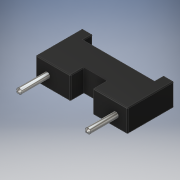
# Autodesk Inventor part: IC_Sockel_2P_2
Saved by Autodesk Inventor 2017 SP1 (Build 210196100, 196)
## iProperties
Part Number: IC_Sockel_2P_2
Material: Generisch
Document SubType Name: Modeling
Designer: Alex
Density: 1 g/cm^3
Appearance: Vorgabe
Author: Alex
Autodesk Inventor part; units mm, degrees
sketch "Skizze1" plane through (0, 0, 0) normal (0, 0, 1) x (1, 0, 0)
  line L0 (0, 0) -> (5.08, 0)
  line L1 (5.08, 0) -> (5.08, 5.16)
  line L2 (5.08, 5.16) -> (0, 5.16)
  line L3 (0, 5.16) -> (0, 0)
  dimension "d0" = 5.08
  dimension "d1" = 5.16
  constraints: 8 end point, 2 parallel, 1 horizontal, 1 perpendicular
  measures "d0" distance of L2.end L1.end
  measures "d1" distance of L1.end L0.end
extrude "Extrusion1" add sketch "Skizze1" against normal blind 2.54
sketch "Skizze2" plane through (0, 0, 0) normal (0, -1, 0) x (1, 0, 0)
  circle A0 centre (3.81, -1.27) radius 0.3
  line L0 (0, 0) -> (0, -2.54) projected
  line L1 (0, -2.54) -> (5.08, -2.54) projected
  dimension "d4" = 0.6
  dimension "d5" = 3.81
  dimension "d7" = 1.27
  constraints: 1 centre point
  measures "d4" diameter of A0
  measures "d5" distance from line of L0 A0.centre
  measures "d7" distance from line of L1 A0.centre
extrude "Extrusion2" add sketch "Skizze2" along normal blind 3.3
sketch "Skizze3" plane through (0, 5.16, 0) normal (0, 1, 0) x (1, 0, 0)
  line L0 (1.935, 2.02) -> (3.935, 2.02)
  line L1 (3.935, 2.02) -> (3.935, 0.52)
  line L2 (3.935, 0.52) -> (1.935, 0.52)
  line L3 (1.935, 0.52) -> (1.935, 2.02)
  line L4 (5.08, 0) -> (5.08, 2.54) projected
  line L5 (5.08, 0) -> (0, 0) projected
  dimension "d10" = 2
  dimension "d11" = 1.5
  dimension "d12" = 1.145
  dimension "d13" = 0.52
  constraints: 8 end point, 2 parallel, 1 horizontal, 1 perpendicular
  measures "d10" distance of L1.end L2.end
  measures "d11" distance of L0.end L1.end
  measures "d12" distance between parallel lines of L4 L1
  measures "d13" distance between parallel lines of L5 L2
extrude "Extrusion3" cut sketch "Skizze3" against normal blind 2
sketch "Skizze4" plane through (0, 3.16, 0) normal (0, 1, 0) x (1, 0, 0)
  line L0 (3.935, 2.02) -> (3.935, 0.52) projected
  line L1 (3.935, 0.52) -> (1.935, 0.52) projected
  line L2 (3.935, 2.02) -> (3.435, 2.02)
  line L3 (3.435, 2.02) -> (3.435, 0.52)
  line L4 (3.435, 0.52) -> (3.935, 0.52)
  line L5 (3.935, 0.52) -> (3.935, 2.02)
  point P0 (0, 0)
  dimension "d16" = 0.5
  constraints: 8 end point, 2 parallel, 1 horizontal, 1 perpendicular, 1 point on line
  measures "d16" distance of L4.end L3.end
extrude "Extrusion4" cut sketch "Skizze4" against normal blind 1
chamfer "Fase1" distance 0.5 angle 45 1 edges at (3.435, 3.16, -1.27)
ref_plane "Arbeitsebene1" through (0, 5.16, -2.54) normal (0, 1, 0) x (1, 0, 0)
ref_plane "Arbeitsebene2" through (0, 0, -2.54) normal (-1, 0, 0) x (0, 0, 1)
fillet "Rundung1" radius 1 1 edges at (2.935, 3.16, -1.27)
fillet "Rundung2" radius 0.5 1 edges at (3.435, 2.66, -1.27)
chamfer "Fase2" distance 0.2 angle 45 1 edges at (3.51, -3.3, -1.27)
mirror "Spiegeln1" about plane through (0, 0, -2.54) normal (-1, 0, 0) of "Extrusion1", "Extrusion2", "Extrusion3", "Extrusion4", "Fase1", "Rundung1", "Rundung2", "Fase2"
pattern_of_one "Rechteckige Anordnung1"
sketch "Skizze5" plane through (0, 5.16, -2.54) normal (0, 1, 0) x (1, 0, 0)
  line L0 (3.935, -2.54) -> (-3.935, -2.54)
  line L1 (-3.935, -2.54) -> (-3.935, 0)
  line L2 (-3.935, 0) -> (3.935, 0)
  line L3 (3.935, 0) -> (3.935, -2.54)
  line L4 (5.08, -2.54) -> (-5.08, -2.54) projected
  line L5 (-3.935, -2.02) -> (-3.935, -0.52) projected
  line L6 (3.935, -0.52) -> (3.935, -2.02) projected
  point P0 (0, -2.54)
  point P1 (0, -2.54)
  dimension "versenkung_Z" = 2.54
  constraints: 8 end point, 2 collinear, 2 midpoint, 2 parallel, 1 perpendicular
  measures "versenkung_Z" distance of L0.end L1.end
extrude "Extrusion5" cut sketch "Skizze5" against normal blind 1
ref_plane "Arbeitsebene3" through (3.935, 0, 0) normal (0, 1, 0) x (1, 0, 0)
sketch "Skizze12" plane through (3.935, 0, 0) normal (0, 1, 0) x (1, 0, 0)
  line L0 (-5.185, 0) -> (-2.685, 0)
  line L1 (-2.685, 0) -> (-2.685, 2.54)
  line L2 (-2.685, 2.54) -> (-5.185, 2.54)
  line L3 (-5.185, 2.54) -> (-5.185, 0)
  line L4 (1.145, 0) -> (0, 0) projected
  point P0 (-3.935, 0)
  dimension "d54" = 2.5
  dimension "d60" = 3.83
  dimension "d61" = 2.54
  constraints: 8 end point, 2 parallel, 1 horizontal, 1 midpoint, 1 perpendicular
  measures "d54" distance of L1.end L2.end
  measures "d60" distance from line of L4.start L1
  measures "d61" distance of L0.end L1.end
extrude "Extrusion8" cut sketch "Skizze12" along normal blind 1.5
fillet "Rundung4" radius 0.1 17 edges at (-5.08, 0, -1.27) (3.165, 0, 0) (-5.08, 2.58, 0) (1.25, 0, -1.27) (1.25, 0.75, 0) (-1.25, 0.75, 0) (-1.25, 0, -1.27) (5.08, 2.58, 0) (5.08, 0, -1.27) (5.08, 5.16, -1.27) (3.935, 5.16, -1.27) (4.5075, 5.16, 0) (3.935, 4.66, 0) (0, 4.16, 0) (-3.935, 4.66, 0) (-3.935, 5.16, -1.27) (-5.08, 5.16, -1.27)
fillet "Rundung24" radius 0.1 13 edges at (5.0507, 5.1307, -2.54) (1.2793, 0.0293, -2.54) (3.165, 0, -2.54) (1.25, 0.8, -2.54) (4.5075, 5.16, -2.54) (3.9643, 5.1307, -2.54) (3.935, 4.61, -2.54) (5.08, 2.58, -2.54) (0, 1.5, -2.54) (-5.08, 2.58, -2.54) (-3.935, 4.6101, -2.54) (-1.25, 0.8, -2.54) (0, 4.16, -2.54)
equation "\"versenkung_Z\" = 2.54 * AnzPinPaare"
equation "\"d61\" = 2.54 * AnzPinPaare"
equation "\"AnzPinPaare\" = 1"
